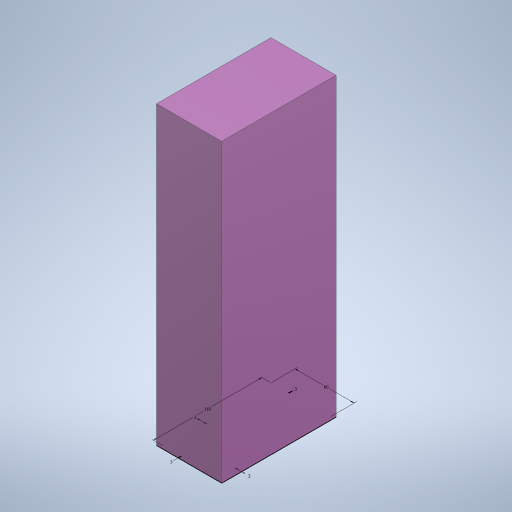
# Autodesk Inventor part: caja
Saved by Autodesk Inventor 2023 (Build 270158000, 158)
## iProperties
Created: 2022-04-26
Part Number: caja
Material: Genérico
Document SubType Name: Modeling
Designer: isaac
Density: 1 g/cm^3
Appearance: Valor por defecto
Author: isaac
Autodesk Inventor part; units mm, degrees
ref_plane "YZ Plane" through (0, 0, 0) normal (1, 0, 0) x (0, 1, 0)
ref_plane "XZ Plane" through (0, 0, 0) normal (0, 1, 0) x (-1, 0, 0)
ref_plane "XY Plane" through (0, 0, 0) normal (0, 0, 1) x (1, 0, 0)
sketch "Boceto1" plane through (0, 0, 0) normal (0, 1, 0) x (-1, 0, 0)
  line L0 (30, 55) -> (-30, 55)
  line L1 (-30, 55) -> (-30, -55)
  line L2 (-30, -55) -> (30, -55)
  line L3 (30, -55) -> (30, 55)
  line L4 (33, 58) -> (-33, 58)
  line L5 (-33, 58) -> (-33, -58)
  line L6 (-33, -58) -> (33, -58)
  line L7 (33, -58) -> (33, 58)
  point P0 (0, 0)
  point P1 (0, -55)
  point P2 (30, 0)
  dimension "d0" = 110
  dimension "d1" = 60
  dimension "d2" = 3
  dimension "d3" = 3
  dimension "d4" = 3
  dimension "d5" = 3
  constraints: 16 end point, 4 parallel, 2 horizontal, 2 midpoint, 2 perpendicular, 1 horizontal alignment, 1 vertical alignment
  measures "d0" distance between parallel lines of L2 L0
  measures "d1" distance between parallel lines of L1 L3
  measures "d2" distance between parallel lines of L3 L7
  measures "d3" distance between parallel lines of L0 L4
  measures "d4" distance between parallel lines of L5 L1
  measures "d5" distance between parallel lines of L6 L2
extrude "Extrusión1" add sketch "Boceto1" along normal blind 300
sketch "Boceto2" plane through (0, 300, 0) normal (0, 1, 0) x (1, 0, 0)
  line L0 (33, -58) -> (33, 58) construction
  line L1 (33, 58) -> (-33, 58) construction
  line L2 (-33, 58) -> (-33, -58) construction
  line L3 (-33, -58) -> (33, -58) construction
  line L4 (-30, -55) -> (-30, 55) construction
  line L5 (-30, 55) -> (30, 55) construction
  line L6 (30, 55) -> (30, -55) construction
  line L7 (30, -55) -> (-30, -55) construction
  line L8 (-30, -55) -> (-30, 55) projected
  line L9 (-30, 55) -> (30, 55)
  line L10 (30, 55) -> (30, 58)
  line L11 (30, 58) -> (-30, 58)
  line L12 (-30, 58) -> (-30, 55)
  point P0 (0, 0)
  constraints: 8 end point, 3 perpendicular, 1 horizontal alignment, 1 point on line
extrude "Extrusión2" cut sketch "Boceto2" against normal blind 295
extrude "Extrusión3" add sketch "Boceto1" along normal blind 5 contours L3 L2 L1 L0
sketch "Boceto4" plane through (30, 300, 55) normal (0, 0, -1) x (-1, 0, 0)
  line L0 (0, -295) -> (60, -295) construction
  line L1 (60, -295) -> (60, 0) construction
  line L2 (0, 0) -> (60, 0) construction
  line L3 (0, -295) -> (0, 0) construction
  line L4 (0, -295) -> (0, 0) projected
  line L5 (60, 0) -> (0, 0)
  line L6 (0, 0) -> (0, -5)
  line L7 (0, -5) -> (60, -5)
  line L8 (60, -5) -> (60, 0)
  point P0 (30, -300)
  dimension "d12" = 5
  constraints: 8 end point, 2 parallel, 1 horizontal, 1 perpendicular, 1 point on line
  measures "d12" distance between parallel lines of L2 L7
extrude "Extrusión4" add sketch "Boceto4" along normal blind 113
